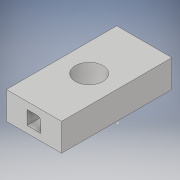
# Autodesk Inventor part: Block
Saved by Autodesk Inventor 2018.2 (Build 222227000, 227)
## iProperties
Created: 2019-01-20
Part Number: Block
Material: Generic
Document SubType Name: Modeling
Designer: faisa
Density: 1 g/cm^3
Appearance: Default
Author: faisa
Autodesk Inventor part; units mm, degrees
ref_plane "YZ Plane" through (0, 0, 0) normal (1, 0, 0) x (0, 1, 0)
ref_plane "XZ Plane" through (0, 0, 0) normal (0, 1, 0) x (-1, 0, 0)
ref_plane "XY Plane" through (0, 0, 0) normal (0, 0, 1) x (1, 0, 0)
sketch "Sketch1" plane through (0, 0, 0) normal (0, 1, 0) x (-1, 0, 0)
  point P0 (0, 0)
sketch "Sketch2" plane through (0, 0, 0) normal (0, 1, 0) x (-1, 0, 0)
  line L0 (52.3958, 50.0021) -> (1.5958, 50.0021)
  line L1 (1.5958, 50.0021) -> (1.5958, -51.5979)
  line L2 (1.5958, -51.5979) -> (52.3958, -51.5979)
  line L3 (52.3958, -51.5979) -> (52.3958, 50.0021)
  circle A0 centre (26.9958, -0.7979) radius 12.7
  point P0 (0, 0)
  dimension "d0" = 101.6
  dimension "d1" = 50.8
  dimension "d2" = 25.4
  dimension "d3" = 50.8
  dimension "d4" = 25.4
  constraints: 8 end point, 2 parallel, 1 centre point, 1 horizontal, 1 perpendicular
  measures "d0" distance of L2.end L0.start
  measures "d1" distance of L0.start L0.end
  measures "d2" diameter of A0
  measures "d3" distance from line of A0.centre L0
  measures "d4" distance from line of A0.centre L3
extrude "Extrusion1" add sketch "Sketch2" along normal blind 25.4
sketch "Sketch4" plane through (-52.3958, 0, 50.0021) normal (0, 0, 1) x (1, 0, 0)
  line L0 (19.05, 19.0241) -> (28.575, 19.0241)
  line L1 (31.75, 15.8491) -> (31.75, 6.3241)
  line L2 (31.75, 6.3241) -> (19.05, 6.3241)
  line L3 (19.05, 6.3241) -> (19.05, 19.0241)
  line L4 (50.8, 0) -> (50.8, 25.4) projected
  line L5 (0, 25.4) -> (50.8, 25.4) projected
  arc A0 (31.75, 15.8491) -> (28.575, 19.0241) centre (28.575, 15.8491) ccw
  point P0 (52.3958, 0)
  point P1 (31.75, 19.0241)
  dimension "d7" = 12.7
  dimension "d8" = 12.7
  dimension "d9" = 19.05
  dimension "d10" = 6.3759
  dimension "d11" = 3.175
  constraints: 8 end point, 2 parallel, 2 point on circle, 2 point on line, 2 tangent, 1 centre point, 1 horizontal, 1 perpendicular
  measures "d7" distance of L0.start point (31.75, 19.024)
  measures "d8" distance of point (31.75, 19.024) L1.end
  measures "d9" distance between parallel lines of L4 L1
  measures "d10" distance between parallel lines of L5 L0
  measures "d11" radius of A0
extrude "Extrusion2" cut sketch "Sketch4" against normal up to next
equation "\"d1\" = 0.5 * d0"
equation "\"d3\" = 0.5 * d0"
body "Solid1"
